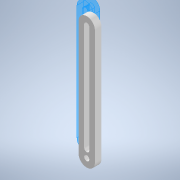
# Autodesk Inventor part: arrow
Saved by Autodesk Inventor 2020 (Build 240168000, 168)
## iProperties
Created: 2022-10-14
Part Number: arrow
Material: Типовые
Document SubType Name: Modeling
Designer: akapu
Density: 1 g/cm^3
Appearance: По умолчанию
Author: akapu
Autodesk Inventor part; units mm, degrees
ref_plane "YZ Plane" through (0, 0, 0) normal (1, 0, 0) x (0, 1, 0)
ref_plane "XZ Plane" through (0, 0, 0) normal (0, 1, 0) x (-1, 0, 0)
ref_plane "XY Plane" through (0, 0, 0) normal (0, 0, 1) x (1, 0, 0)
sketch "Эскиз1" plane through (0, 0, 0) normal (0, 0, 1) x (1, 0, 0)
  line L0 (0, 0) -> (0, 80)
  line L1 (0, 0) -> (0, 5)
  line L2 (0, 80) -> (0, 75)
  circle A0 centre (0, 75) radius 5
  circle A1 centre (0, 5) radius 5
  circle A2 centre (0, 5) radius 1.6
  circle A3 centre (0, 75) radius 1.6
  line L3 (-1.6, 75) -> (-1.6, 5)
  line L4 (1.6, 5) -> (1.6, 75)
  line L5 (-5, 75) -> (-5, 5)
  line L6 (5, 5) -> (5, 75)
  line L7 (-1.6, 9.7371) -> (1.6, 9.7371)
  circle A4 centre (0, 9.7371) radius 1.6
  point P0 (-1.6, 9.7371)
  dimension "d0" = 80
  dimension "d1" = 5
  dimension "d2" = 5
  dimension "d3" = 3.2
  dimension "d4" = 3.2
  constraints: 16 end point, 12 point on circle, 6 tangent, 4 centre point, 4 coincident, 4 point on line, 2 vertical, 1 midpoint, 3 other
  measures "d0" distance of L0.start L0.end
  measures "d1" distance of L0.start L1.end
  measures "d2" distance of L0.end L2.end
  measures "d3" diameter of A2
  measures "d4" diameter of A3
extrude "Выдавливание1" add sketch "Эскиз1" along normal blind 55 contours A1 L3 A2 L0 | L0 A2 L4 A1 | L5 A0 L3 A1 | A1 L4 A0 L6 | L3 A4 L0 A2 | A2 L0 A4 L4 | A0 L0 A3 L3 | A0 L4 A3 L0 picked at (-1.9727, 72.0221) picked at (1.9727, 72.0221)
ref_plane "РабПлоскость1" through (0, 0, 27.5) normal (0, 0, -1) x (-1, 0, 0)
sketch "Эскиз2" plane through (0, 0, 27.5) normal (0, 0, -1) x (-1, 0, 0)
  circle A0 centre (0, 5) radius 1.6 projected
  circle A1 centre (0, 5) radius 5
  line L0 (-5, 5) -> (-5, 75) projected
  ellipse E0 centre (0, 5) end of major axis (-5, 5) minor radius 3.1371
  line L1 (5, 75) -> (5, 5) projected
  line L2 (5, 5) -> (-5, 5)
  line L3 (-5, 5) -> (-5, 83.8736)
  line L4 (-5, 83.8736) -> (5, 83.8736)
  line L5 (5, 83.8736) -> (5, 5)
  point P0 (0, 0)
  constraints: 8 end point, 2 coincident, 2 parallel, 1 centre point, 1 horizontal, 1 perpendicular, 1 point on circle, 1 vertical, 3 other
extrude "Выдавливание2" cut sketch "Эскиз2" against normal mid plane 47 contours E0 A1 | A1 L0 L3 L4 L5 L1 picked at (-0.9942, 8.9185)
